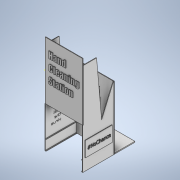
# Autodesk Inventor part: hand-cleaning-body
Saved by Autodesk Inventor 2020.2 (Build 242310000, 310)
## iProperties
Created: 2020-03-25
Part Number: hand-cleaning-body
Material: Generic
Document SubType Name: Modeling
Designer: iamin
Density: 1 g/cm^3
Appearance: Default
Author: iamin
Autodesk Inventor part; units mm, degrees
(part 1 of 2)
ref_plane "YZ Plane" through (0, 0, 0) normal (1, 0, 0) x (0, 1, 0)
ref_plane "XY Plane" through (0, 0, 0) normal (0, 0, 1) x (1, 0, 0)
sketch "Sketch1" plane through (0, 0, 0) normal (0, 0, 1) x (1, 0, 0)
  line L0 (-45.3, -70) -> (45.3, -70)
  line L1 (45.3, -70) -> (45.3, 70)
  line L2 (45.3, 70) -> (-45.3, 70)
  line L3 (-45.3, 70) -> (-45.3, -70)
  line L4 (-45.3, -70) -> (45.3, 70) construction
  line L5 (45.3, -70) -> (-45.3, 70) construction
  point P0 (0, 0)
  dimension "topsize" = 90.6
  dimension "d1" = 140
  constraints: 12 end point, 2 midpoint, 2 parallel, 1 horizontal, 1 perpendicular
  measures "topsize" distance of L2.end L1.end
  measures "d1" distance of L1.end L0.end
extrude "Extrusion1" add sketch "Sketch1" along normal mid plane 1.3
sketch "Sketch2" plane through (45.3, -70, 0.65) normal (1, 0, 0) x (0, 0, -1)
  line L0 (1.3, 125.1437) -> (33.3, 125.1437)
  line L1 (-0.1992, -99) -> (140.3032, -99)
  line L2 (1.3, 0) -> (0, 0) projected
  line L3 (75.8394, -99) -> (75.8394, 14.3341)
  line L4 (1.3, 140) -> (1.3, 0) projected
  line L5 (33.3, 125.1437) -> (45.5649, -11.2927)
  line L6 (74.2941, 54.8516) -> (45.5649, -11.2927)
  line L7 (75.8394, 14.3341) -> (75.8394, 54.8516)
  line L8 (75.8394, 54.8516) -> (74.2941, 54.8516)
  line L9 (-0.1992, 0) -> (-0.1992, -99)
  line L10 (0.65, 0) -> (-0.1992, 0)
  point P0 (0.65, 70)
  dimension "d4" = 99
  dimension "d5" = 74.5394
  dimension "d7" = 32
  constraints: 18 end point, 3 horizontal, 3 vertical, 2 point on line, 1 midpoint, 1 perpendicular
  measures "d4" distance between parallel lines of L1 L2
  measures "d5" distance from line of L3 L2.start
  measures "d7" distance of L0.start L0.end
extrude "Extrusion2" add sketch "Sketch2" along normal mid plane 1.3
mirror "Mirror1" about plane through (0, 0, 0) normal (1, 0, 0) of "Extrusion2"
sketch "Sketch3" plane through (-45.95, -169, -75.1894) normal (-1, 0, 0) x (0, 0, 1)
  point P0 (75.1894, 169)
sketch "Sketch4" plane through (45.95, -169, -75.1894) normal (0, 0, -1) x (-1, 0, 0)
  line L0 (-0.1836, 153.786) -> (91.9029, 153.786)
  line L1 (91.9029, 153.786) -> (91.9029, 0.1386)
  line L2 (91.9029, 0.1386) -> (-0.1836, 0.1386)
  line L3 (-0.1836, 0.1386) -> (-0.1836, 153.786)
  point P0 (45.95, 169)
  constraints: 8 end point, 2 parallel, 1 horizontal, 1 perpendicular
extrude "Extrusion3" add sketch "Sketch4" along normal mid plane 1.3
sketch "Sketch5" plane through (-45.95, -70, -0.65) normal (-1, 0, 0) x (0, 0, 1)
  line L0 (-75.2386, -98.82) -> (-124.9776, -98.82)
  line L1 (-75.2386, -96.5831) -> (-124.9776, -96.5831)
  line L2 (-124.9776, -96.5831) -> (-124.9776, -98.82)
  line L3 (-75.2386, -96.5831) -> (-75.2386, -98.82)
  point P0 (0.65, 70)
  constraints: 8 end point, 2 horizontal, 1 perpendicular, 1 vertical
extrude "Extrusion4" add sketch "Sketch5" against normal blind 91.9
sketch "Sketch6" plane through (-45.95, -70, -0.65) normal (-1, 0, 0) x (0, 0, 1)
  point P0 (0.65, 70)
sketch "Sketch7" plane through (-44.65, -169, 0.8492) normal (0, 0, 1) x (1, 0, 0)
  line L0 (0, 24.5) -> (1.5, 24.5)
  line L1 (1.5, 24.5) -> (1.5, 26)
  line L2 (1.5, 26) -> (0, 26)
  line L3 (0, 0) -> (1.5, 0)
  line L4 (1.5, 0) -> (1.5, 1.5)
  line L5 (1.5, 1.5) -> (0, 1.5)
  line L6 (0, 26) -> (0, 0)
  point P0 (44.65, 169)
  point P1 (0, 24.5)
  point P2 (0, 1.5)
  dimension "d15" = 1.5
  dimension "d16" = 1.5
  dimension "d17" = 1.5
  dimension "d18" = 1.5
  dimension "d19" = 26
  constraints: 14 end point, 4 perpendicular, 2 horizontal, 1 vertical
  measures "d15" distance of L0.start L0.end
  measures "d16" distance of L3.start L3.end
  measures "d17" distance of L3.end L4.end
  measures "d18" distance of L1.end L0.end
  measures "d19" distance of L1.end L3.end
extrude "Extrusion5" add sketch "Sketch7" against normal blind 74.5394
mirror "Mirror2" about plane through (0, 0, 0) normal (1, 0, 0) of "Extrusion5"
sketch "Sketch8" plane through (-44.65, -70, -0.65) normal (0, -1, 0) x (1, 0, 0)
  line L0 (0, 0) -> (44.65, 0)
  line L1 (44.65, -41.1247) -> (0, -41.1247)
  line L2 (0, -41.1247) -> (0, 0)
  line L3 (89.3, 0) -> (44.65, 0)
  line L4 (44.65, -41.1247) -> (89.3, -41.1247)
  line L5 (89.3, -41.1247) -> (89.3, 0)
  point P0 (44.65, 0.65)
  constraints: 12 end point, 1 horizontal, 1 parallel
extrude "Extrusion6" [suppressed]
sketch "Sketch10" plane through (-45.9529, -15.214, -75.8394) normal (0, 1, 0) x (1, 0, 0)
  line L0 (58.8396, -1.3) -> (58.8396, -5.46)
  line L1 (58.8396, -5.46) -> (55.5586, -5.46)
  line L2 (55.5586, -5.46) -> (55.5586, -4.16)
  line L3 (55.5586, -4.16) -> (57.5396, -4.16)
  line L4 (57.5396, -4.16) -> (57.5396, -1.3)
  line L5 (90.6029, -1.3) -> (1.3029, -1.3) projected
  line L6 (45.9529, 0.1482) -> (45.9529, -6.4647)
  line L7 (58.8396, -1.3) -> (57.5396, -1.3)
  line L8 (33.0662, -1.3) -> (33.0662, -5.46)
  line L9 (33.0662, -5.46) -> (36.3472, -5.46)
  line L10 (36.3472, -5.46) -> (36.3472, -4.16)
  line L11 (36.3472, -4.16) -> (34.3662, -4.16)
  line L12 (34.3662, -4.16) -> (34.3662, -1.3)
  line L13 (1.3029, -1.3) -> (90.6029, -1.3)
  line L14 (33.0662, -1.3) -> (34.3662, -1.3)
  point P0 (45.9529, -75.8394)
  dimension "d25" = 1.3
  dimension "d26" = 1.3
  dimension "d27" = 2.86
  constraints: 28 end point, 8 symmetric about line, 3 perpendicular, 2 horizontal, 2 vertical, 1 point on line
  measures "d25" distance between parallel lines of L0 L4
  measures "d26" distance between parallel lines of L1 L3
  measures "d27" distance between parallel lines of L5 L3
extrude "Extrusion7" [suppressed]
sketch "Sketch11" plane through (0, 0, 0.65) normal (0, 0, 1) x (1, 0, 0)
  line L0 (-36.7165, 46.3764) -> (38.2753, 46.3764) construction
  line L1 (38.2753, 46.3764) -> (38.2753, 2.6535) construction
  line L2 (38.2753, 2.6535) -> (-36.7165, 2.6535) construction
  line L3 (-36.7165, 2.6535) -> (-36.7165, 46.3764) construction
  line L4 (-26.2582, 46.3764) -> (-26.2582, 30.2764)
  line L5 (-26.2582, 30.2764) -> (-30.444, 30.2764)
  line L6 (-30.444, 30.2764) -> (-30.444, 37.0343)
  line L7 (-30.444, 37.0343) -> (-31.6936, 37.0343)
  line L8 (-31.6936, 37.0343) -> (-31.6936, 30.2764)
  line L9 (-31.6936, 30.2764) -> (-35.8794, 30.2764)
  line L10 (-35.8794, 30.2764) -> (-35.8794, 46.3764)
  line L11 (-35.8794, 46.3764) -> (-31.6936, 46.3764)
  line L12 (-31.6936, 46.3764) -> (-31.6936, 40.6134)
  line L13 (-31.6936, 40.6134) -> (-30.444, 40.6134)
  line L14 (-30.444, 40.6134) -> (-30.444, 46.3764)
  line L15 (-30.444, 46.3764) -> (-26.2582, 46.3764)
  line L16 (-21.1018, 38.3689) -> (-24.8751, 38.3689)
  line L17 (-24.8751, 38.3689) -> (-24.8751, 39.2546)
  spline S0 degree 2 poles (-24.8751, 39.2546) (-24.8751, 40.7833) (-24.1714, 42.4455) (-22.036, 43.7194) (-20.3375, 43.7194) knots 0 0 0 1 2 3 3 3
  spline S1 degree 2 poles (-20.3375, 43.7194) (-18.2992, 43.7194) (-16.2245, 42.2756) (-15.812, 40.1767) (-15.812, 36.9009) knots 0 0 0 1 2 3 3 3
  line L18 (-15.812, 36.9009) -> (-15.812, 30.2764)
  line L19 (-15.812, 30.2764) -> (-19.7187, 30.2764)
  line L20 (-19.7187, 30.2764) -> (-19.7187, 31.4533)
  spline S2 degree 2 poles (-19.7187, 31.4533) (-20.0827, 30.7496) (-21.2474, 30.0338) (-22.0603, 30.0338) knots 0 0 0 1 2 2 2
  spline S3 degree 2 poles (-22.0603, 30.0338) (-23.1158, 30.0338) (-24.8751, 31.2228) (-24.8751, 33.2247) knots 0 0 0 1 2 2 2
  line L21 (-24.8751, 33.2247) -> (-24.8751, 34.3045)
  spline S4 degree 2 poles (-24.8751, 34.3045) (-24.8751, 35.7847) (-23.9409, 36.8645) (-22.0846, 37.5803) knots 0 0 0 1 2 2 2
  spline S5 degree 2 poles (-22.0846, 37.5803) (-20.107, 38.3568) (-19.8279, 38.8906) (-19.8279, 39.7156) knots 0 0 0 1 2 2 2
  spline S6 degree 2 poles (-19.8279, 39.7156) (-19.8279, 40.7469) (-20.1312, 41.3778) (-20.4952, 41.3778) knots 0 0 0 1 2 2 2
  spline S7 degree 2 poles (-20.4952, 41.3778) (-20.9077, 41.3778) (-21.1018, 40.8561) (-21.1018, 39.752) knots 0 0 0 1 2 2 2
  line L22 (-21.1018, 39.752) -> (-21.1018, 38.3689)
  spline S8 degree 2 poles (-19.8279, 36.5612) (-20.7985, 35.8575) (-21.1018, 34.899) (-21.1018, 34.0012) knots 0 0 0 1 2 2 2
  spline S9 degree 2 poles (-21.1018, 34.0012) (-21.1018, 32.9699) (-20.8349, 32.3754) (-20.4345, 32.3754) knots 0 0 0 1 2 2 2
  spline S10 degree 2 poles (-20.4345, 32.3754) (-20.0584, 32.3754) (-19.8279, 32.8486) (-19.8279, 33.8434) knots 0 0 0 1 2 2 2
  line L23 (-19.8279, 33.8434) -> (-19.8279, 36.5612)
  line L24 (-10.3402, 43.4767) -> (-10.413, 42.2635)
  spline S11 degree 2 poles (-10.413, 42.2635) (-9.9762, 42.9914) (-8.7144, 43.7194) (-7.8894, 43.7194) knots 0 0 0 1 2 2 2
  spline S12 degree 2 poles (-7.8894, 43.7194) (-6.846, 43.7194) (-5.5357, 42.7488) (-5.1596, 41.2565) (-5.1596, 39.5336) knots 0 0 0 1 2 3 3 3
  line L25 (-5.1596, 39.5336) -> (-5.1596, 30.2764)
  line L26 (-5.1596, 30.2764) -> (-9.1755, 30.2764)
  line L27 (-9.1755, 30.2764) -> (-9.1755, 39.4123)
  spline S13 degree 2 poles (-9.1755, 39.4123) (-9.1755, 40.7833) (-9.3574, 41.3778) (-9.77, 41.3778) knots 0 0 0 1 2 2 2
  spline S14 degree 2 poles (-9.77, 41.3778) (-10.1946, 41.3778) (-10.413, 40.6862) (-10.413, 39.1939) knots 0 0 0 1 2 2 2
  line L28 (-10.413, 39.1939) -> (-10.413, 30.2764)
  line L29 (-10.413, 30.2764) -> (-14.4289, 30.2764)
  line L30 (-14.4289, 30.2764) -> (-14.4289, 43.4767)
  line L31 (-14.4289, 43.4767) -> (-10.3402, 43.4767)
  line L32 (5.3594, 46.3764) -> (5.3594, 30.2764)
  line L33 (5.3594, 30.2764) -> (1.3435, 30.2764)
  line L34 (1.3435, 30.2764) -> (1.3435, 31.2349)
  spline S15 degree 2 poles (1.3435, 31.2349) (0.7612, 30.6283) (-0.5006, 30.0338) (-1.2043, 30.0338) knots 0 0 0 1 2 2 2
  spline S16 degree 2 poles (-1.2043, 30.0338) (-2.1385, 30.0338) (-3.5095, 31.0165) (-3.8978, 32.3147) (-3.8978, 33.7706) knots 0 0 0 1 2 3 3 3
  line L35 (-3.8978, 33.7706) -> (-3.8978, 39.9583)
  spline S17 degree 2 poles (-3.8978, 39.9583) (-3.8978, 41.4749) (-3.5095, 42.7488) (-2.1143, 43.7194) (-1.1558, 43.7194) knots 0 0 0 1 2 3 3 3
  spline S18 degree 2 poles (-1.1558, 43.7194) (-0.4036, 43.7194) (0.834, 43.1856) (1.3435, 42.6396) knots 0 0 0 1 2 2 2
  line L36 (1.3435, 42.6396) -> (1.3435, 46.3764)
  line L37 (1.3435, 46.3764) -> (5.3594, 46.3764)
  spline S19 degree 2 poles (1.3435, 40.1524) (1.3435, 40.8804) (1.0888, 41.3778) (0.7248, 41.3778) knots 0 0 0 1 2 2 2
  spline S20 degree 2 poles (0.7248, 41.3778) (0.3729, 41.3778) (0.1181, 40.9289) (0.1181, 40.1524) knots 0 0 0 1 2 2 2
  line L38 (0.1181, 40.1524) -> (0.1181, 33.6857)
  spline S21 degree 2 poles (0.1181, 33.6857) (0.1181, 32.885) (0.3608, 32.3754) (0.7005, 32.3754) knots 0 0 0 1 2 2 2
  spline S22 degree 2 poles (0.7005, 32.3754) (1.0888, 32.3754) (1.3435, 32.9456) (1.3435, 34.0497) knots 0 0 0 1 2 2 2
  line L39 (1.3435, 34.0497) -> (1.3435, 40.1524)
  line L40 (-26.1005, 12.4203) -> (-30.2862, 12.4203)
  line L41 (-30.2862, 12.4203) -> (-30.2862, 15.2229)
  spline S23 degree 2 poles (-30.2862, 15.2229) (-30.2862, 16.4362) (-30.5531, 17.0428) (-31.0142, 17.0428) knots 0 0 0 1 2 2 2
  spline S24 degree 2 poles (-31.0142, 17.0428) (-31.5359, 17.0428) (-31.8149, 16.3027) (-31.8149, 15.0895) knots 0 0 0 1 2 2 2
  line L42 (-31.8149, 15.0895) -> (-31.8149, 7.6158)
  spline S25 degree 2 poles (-31.8149, 7.6158) (-31.8149, 6.4389) (-31.5359, 5.7231) (-31.0506, 5.7231) knots 0 0 0 1 2 2 2
  spline S26 degree 2 poles (-31.0506, 5.7231) (-30.5774, 5.7231) (-30.2862, 6.4389) (-30.2862, 7.7614) knots 0 0 0 1 2 2 2
  line L43 (-30.2862, 7.7614) -> (-30.2862, 9.7875)
  line L44 (-30.2862, 9.7875) -> (-26.1005, 9.7875)
  line L45 (-26.1005, 9.7875) -> (-26.1005, 9.1566)
  spline S27 degree 2 poles (-26.1005, 9.1566) (-26.1005, 6.6573) (-26.8042, 4.5705) (-29.2307, 2.9932) (-30.9899, 2.9932) knots 0 0 0 1 2 3 3 3
  spline S28 degree 2 poles (-30.9899, 2.9932) (-32.8341, 2.9932) (-35.2242, 4.3278) (-36.0007, 6.6816) (-36.0007, 9.0474) knots 0 0 0 1 2 3 3 3
  line L46 (-36.0007, 9.0474) -> (-36.0007, 13.7549)
  spline S29 degree 2 poles (-36.0007, 13.7549) (-36.0007, 15.4898) (-35.758, 17.2369) (-34.5812, 18.8506) (-32.4822, 19.7727) (-31.1112, 19.7727) knots 0 0 0 1 2 3 4 4 4
  spline S30 degree 2 poles (-31.1112, 19.7727) (-29.2671, 19.7727) (-26.8527, 18.341) (-26.1005, 16.2057) (-26.1005, 13.949) knots 0 0 0 1 2 3 3 3
  line L47 (-26.1005, 13.949) -> (-26.1005, 12.4203)
  line L48 (-20.5801, 19.4329) -> (-20.5801, 3.3329)
  line L49 (-20.5801, 3.3329) -> (-24.7174, 3.3329)
  line L50 (-24.7174, 3.3329) -> (-24.7174, 19.4329)
  line L51 (-24.7174, 19.4329) -> (-20.5801, 19.4329)
  line L52 (-10.0369, 9.7026) -> (-15.2418, 9.7026)
  line L53 (-15.2418, 9.7026) -> (-15.2418, 6.8514)
  spline S31 degree 2 poles (-15.2418, 6.8514) (-15.2418, 5.9536) (-14.987, 5.4319) (-14.6109, 5.4319) knots 0 0 0 1 2 2 2
  spline S32 degree 2 poles (-14.6109, 5.4319) (-14.1498, 5.4319) (-13.8465, 6.1235) (-13.8465, 7.1062) knots 0 0 0 1 2 2 2
  line L54 (-13.8465, 7.1062) -> (-13.8465, 8.8412)
  line L55 (-13.8465, 8.8412) -> (-10.0369, 8.8412)
  line L56 (-10.0369, 8.8412) -> (-10.0369, 7.8705)
  spline S33 degree 2 poles (-10.0369, 7.8705) (-10.0369, 6.6452) (-10.3402, 5.3348) (-11.4807, 3.8425) (-13.2156, 3.0903) (-14.5381, 3.0903) knots 0 0 0 1 2 3 4 4 4
  spline S34 degree 2 poles (-14.5381, 3.0903) (-15.812, 3.0903) (-17.7532, 3.8304) (-18.8452, 5.1164) (-19.2577, 6.6573) (-19.2577, 8.1253) knots 0 0 0 1 2 3 4 4 4
  line L57 (-19.2577, 8.1253) -> (-19.2577, 11.9835)
  spline S35 degree 2 poles (-19.2577, 11.9835) (-19.2577, 13.7063) (-18.3235, 15.7082) (-16.1881, 16.7759) (-14.8171, 16.7759) knots 0 0 0 1 2 3 3 3
  spline S36 degree 2 poles (-14.8171, 16.7759) (-13.1186, 16.7759) (-10.9226, 15.4898) (-10.0369, 13.3788) (-10.0369, 11.4497) knots 0 0 0 1 2 3 3 3
  line L58 (-10.0369, 11.4497) -> (-10.0369, 9.7026)
  line L59 (-14.0649, 11.8501) -> (-14.0649, 12.8085)
  spline S37 degree 2 poles (-14.0649, 12.8085) (-14.0649, 13.8398) (-14.2833, 14.4343) (-14.623, 14.4343) knots 0 0 0 1 2 2 2
  spline S38 degree 2 poles (-14.623, 14.4343) (-15.0476, 14.4343) (-15.2418, 13.9247) (-15.2418, 12.8085) knots 0 0 0 1 2 2 2
  line L60 (-15.2418, 12.8085) -> (-15.2418, 11.8501)
  line L61 (-15.2418, 11.8501) -> (-14.0649, 11.8501)
  line L62 (-5.1353, 11.4254) -> (-8.9085, 11.4254)
  line L63 (-8.9085, 11.4254) -> (-8.9085, 12.3111)
  spline S39 degree 2 poles (-8.9085, 12.3111) (-8.9085, 13.8398) (-8.2048, 15.502) (-6.0695, 16.7759) (-4.3709, 16.7759) knots 0 0 0 1 2 3 3 3
  spline S40 degree 2 poles (-4.3709, 16.7759) (-2.3327, 16.7759) (-0.258, 15.3321) (0.1545, 13.2332) (0.1545, 9.9574) knots 0 0 0 1 2 3 3 3
  line L64 (0.1545, 9.9574) -> (0.1545, 3.3329)
  line L65 (0.1545, 3.3329) -> (-3.7522, 3.3329)
  line L66 (-3.7522, 3.3329) -> (-3.7522, 4.5098)
  spline S41 degree 2 poles (-3.7522, 4.5098) (-4.1161, 3.8061) (-5.2809, 3.0903) (-6.0938, 3.0903) knots 0 0 0 1 2 2 2
  spline S42 degree 2 poles (-6.0938, 3.0903) (-7.1493, 3.0903) (-8.9085, 4.2793) (-8.9085, 6.2812) knots 0 0 0 1 2 2 2
  line L67 (-8.9085, 6.2812) -> (-8.9085, 7.361)
  spline S43 degree 2 poles (-8.9085, 7.361) (-8.9085, 8.8412) (-7.9743, 9.921) (-6.118, 10.6368) knots 0 0 0 1 2 2 2
  spline S44 degree 2 poles (-6.118, 10.6368) (-4.1404, 11.4133) (-3.8614, 11.9471) (-3.8614, 12.7721) knots 0 0 0 1 2 2 2
  spline S45 degree 2 poles (-3.8614, 12.7721) (-3.8614, 13.8034) (-4.1647, 14.4343) (-4.5287, 14.4343) knots 0 0 0 1 2 2 2
  spline S46 degree 2 poles (-4.5287, 14.4343) (-4.9412, 14.4343) (-5.1353, 13.9126) (-5.1353, 12.8085) knots 0 0 0 1 2 2 2
  line L68 (-5.1353, 12.8085) -> (-5.1353, 11.4254)
  spline S47 degree 2 poles (-3.8614, 9.6176) (-4.832, 8.914) (-5.1353, 7.9555) (-5.1353, 7.0577) knots 0 0 0 1 2 2 2
  spline S48 degree 2 poles (-5.1353, 7.0577) (-5.1353, 6.0264) (-4.8684, 5.4319) (-4.468, 5.4319) knots 0 0 0 1 2 2 2
  spline S49 degree 2 poles (-4.468, 5.4319) (-4.0919, 5.4319) (-3.8614, 5.9051) (-3.8614, 6.8999) knots 0 0 0 1 2 2 2
  line L69 (-3.8614, 6.8999) -> (-3.8614, 9.6176)
  line L70 (5.6264, 16.5332) -> (5.5536, 15.32)
  spline S50 degree 2 poles (5.5536, 15.32) (5.9903, 16.0479) (7.2521, 16.7759) (8.0771, 16.7759) knots 0 0 0 1 2 2 2
  spline S51 degree 2 poles (8.0771, 16.7759) (9.1206, 16.7759) (10.4309, 15.8053) (10.807, 14.313) (10.807, 12.5901) knots 0 0 0 1 2 3 3 3
  line L71 (10.807, 12.5901) -> (10.807, 3.3329)
  line L72 (10.807, 3.3329) -> (6.7911, 3.3329)
  line L73 (6.7911, 3.3329) -> (6.7911, 12.4688)
  spline S52 degree 2 poles (6.7911, 12.4688) (6.7911, 13.8398) (6.6091, 14.4343) (6.1966, 14.4343) knots 0 0 0 1 2 2 2
  spline S53 degree 2 poles (6.1966, 14.4343) (5.7719, 14.4343) (5.5536, 13.7427) (5.5536, 12.2504) knots 0 0 0 1 2 2 2
  line L74 (5.5536, 12.2504) -> (5.5536, 3.3329)
  line L75 (5.5536, 3.3329) -> (1.5377, 3.3329)
  line L76 (1.5377, 3.3329) -> (1.5377, 16.5332)
  line L77 (1.5377, 16.5332) -> (5.6264, 16.5332)
  line L78 (16.3273, 16.5332) -> (16.3273, 3.3329)
  line L79 (16.3273, 3.3329) -> (12.1901, 3.3329)
  line L80 (12.1901, 3.3329) -> (12.1901, 16.5332)
  line L81 (12.1901, 16.5332) -> (16.3273, 16.5332)
  line L82 (16.3273, 19.4329) -> (16.3273, 17.334)
  line L83 (16.3273, 17.334) -> (12.1901, 17.334)
  line L84 (12.1901, 17.334) -> (12.1901, 19.4329)
  line L85 (12.1901, 19.4329) -> (16.3273, 19.4329)
  line L86 (21.8598, 16.5332) -> (21.787, 15.32)
  spline S54 degree 2 poles (21.787, 15.32) (22.2238, 16.0479) (23.4856, 16.7759) (24.3106, 16.7759) knots 0 0 0 1 2 2 2
  spline S55 degree 2 poles (24.3106, 16.7759) (25.354, 16.7759) (26.6643, 15.8053) (27.0404, 14.313) (27.0404, 12.5901) knots 0 0 0 1 2 3 3 3
  line L87 (27.0404, 12.5901) -> (27.0404, 3.3329)
  line L88 (27.0404, 3.3329) -> (23.0245, 3.3329)
  line L89 (23.0245, 3.3329) -> (23.0245, 12.4688)
  spline S56 degree 2 poles (23.0245, 12.4688) (23.0245, 13.8398) (22.8426, 14.4343) (22.43, 14.4343) knots 0 0 0 1 2 2 2
  spline S57 degree 2 poles (22.43, 14.4343) (22.0054, 14.4343) (21.787, 13.7427) (21.787, 12.2504) knots 0 0 0 1 2 2 2
  line L90 (21.787, 12.2504) -> (21.787, 3.3329)
  line L91 (21.787, 3.3329) -> (17.7711, 3.3329)
  line L92 (17.7711, 3.3329) -> (17.7711, 16.5332)
  line L93 (17.7711, 16.5332) -> (21.8598, 16.5332)
  line L94 (37.5594, 16.5332) -> (37.5594, 6.3661)
  spline S58 degree 2 poles (37.5594, 6.3661) (37.5594, 4.3036) (37.3653, 3.1024) (36.2127, 1.7557) (34.1502, 1.052) (32.5972, 1.052) knots 0 0 0 1 2 3 4 4 4
  spline S59 degree 2 poles (32.5972, 1.052) (30.6681, 1.052) (28.3386, 2.3502) (28.3022, 4.2672) knots 0 0 0 1 2 2 2
  line L95 (28.3022, 4.2672) -> (32.1968, 4.2672)
  spline S60 degree 2 poles (32.1968, 4.2672) (32.1968, 3.3936) (32.8398, 3.3936) knots 0 0 0 1 1 1
  spline S61 degree 2 poles (32.8398, 3.3936) (33.3009, 3.3936) (33.6042, 3.9274) (33.6042, 4.7889) knots 0 0 0 1 2 2 2
  line L96 (33.6042, 4.7889) -> (33.6042, 5.7837)
  spline S62 degree 2 poles (33.6042, 5.7837) (33.0825, 5.3106) (31.942, 4.8374) (31.3111, 4.8374) knots 0 0 0 1 2 2 2
  spline S63 degree 2 poles (31.3111, 4.8374) (30.2313, 4.8374) (28.8239, 5.7109) (28.3022, 7.1305) (28.3022, 8.4529) knots 0 0 0 1 2 3 3 3
  line L97 (28.3022, 8.4529) -> (28.3022, 13.2453)
  spline S64 degree 2 poles (28.3022, 13.2453) (28.3022, 15.1259) (29.6611, 16.7759) (31.0442, 16.7759) knots 0 0 0 1 2 2 2
  spline S65 degree 2 poles (31.0442, 16.7759) (31.7964, 16.7759) (33.0461, 16.1571) (33.5314, 15.5384) knots 0 0 0 1 2 2 2
  line L98 (33.5314, 15.5384) -> (33.8226, 16.5332)
  line L99 (33.8226, 16.5332) -> (37.5594, 16.5332)
  spline S66 degree 2 poles (33.5314, 13.0269) (33.5314, 13.9369) (33.3251, 14.4343) (32.9612, 14.4343) knots 0 0 0 1 2 2 2
  spline S67 degree 2 poles (32.9612, 14.4343) (32.6093, 14.4343) (32.3181, 13.8641) (32.3181, 13.0269) knots 0 0 0 1 2 2 2
  line L100 (32.3181, 13.0269) -> (32.3181, 8.5864)
  spline S68 degree 2 poles (32.3181, 8.5864) (32.3181, 7.7007) (32.5365, 7.179) (32.8884, 7.179) knots 0 0 0 1 2 2 2
  spline S69 degree 2 poles (32.8884, 7.179) (33.2888, 7.179) (33.5314, 7.822) (33.5314, 8.9382) knots 0 0 0 1 2 2 2
  line L101 (33.5314, 8.9382) -> (33.5314, 13.0269)
  line L102 (-27.0104, -12.3757) -> (-30.905, -12.3757)
  line L103 (-30.905, -12.3757) -> (-30.905, -11.1867)
  spline S70 degree 2 poles (-30.905, -11.1867) (-30.905, -10.3617) (-31.1962, -9.9007) (-31.548, -9.9007) knots 0 0 0 1 2 2 2
  spline S71 degree 2 poles (-31.548, -9.9007) (-31.9241, -9.9007) (-32.3124, -10.5194) (-32.3124, -11.1382) knots 0 0 0 1 2 2 2
  spline S72 degree 2 poles (-32.3124, -11.1382) (-32.3124, -11.939) (-32.094, -12.3515) knots 0 0 0 1 1 1
  spline S73 degree 2 poles (-32.094, -12.3515) (-31.8756, -12.764) (-30.905, -13.3342) knots 0 0 0 1 1 1
  spline S74 degree 2 poles (-30.905, -13.3342) (-28.1145, -14.9964) (-27.3865, -16.0641) knots 0 0 0 1 1 1
  spline S75 degree 2 poles (-27.3865, -16.0641) (-26.6586, -17.1317) (-26.6586, -19.4976) knots 0 0 0 1 1 1
  spline S76 degree 2 poles (-26.6586, -19.4976) (-26.6586, -21.2204) (-27.4593, -22.8462) (-29.7767, -23.9503) (-31.3054, -23.9503) knots 0 0 0 1 2 3 3 3
  spline S77 degree 2 poles (-31.3054, -23.9503) (-32.9797, -23.9503) (-35.3577, -22.6763) (-36.0978, -20.7109) (-36.0978, -18.9031) knots 0 0 0 1 2 3 3 3
  line L104 (-36.0978, -18.9031) -> (-36.0978, -17.8476)
  line L105 (-36.0978, -17.8476) -> (-32.2032, -17.8476)
  line L106 (-32.2032, -17.8476) -> (-32.2032, -19.8009)
  spline S78 degree 2 poles (-32.2032, -19.8009) (-32.2032, -20.6987) (-31.8756, -21.2204) (-31.4631, -21.2204) knots 0 0 0 1 2 2 2
  spline S79 degree 2 poles (-31.4631, -21.2204) (-31.0385, -21.2204) (-30.6381, -20.5653) (-30.6381, -19.9222) knots 0 0 0 1 2 2 2
  spline S80 degree 2 poles (-30.6381, -19.9222) (-30.6381, -18.5027) (-31.0263, -18.0659) knots 0 0 0 1 1 1
  spline S81 degree 2 poles (-31.0263, -18.0659) (-31.4267, -17.6292) (-32.9918, -16.5979) knots 0 0 0 1 1 1
  spline S82 degree 2 poles (-32.9918, -16.5979) (-34.5448, -15.5666) (-35.5639, -14.6324) (-36.2312, -12.9824) (-36.2312, -11.6963) knots 0 0 0 1 2 3 3 3
  spline S83 degree 2 poles (-36.2312, -11.6963) (-36.2312, -9.84) (-35.2849, -8.1293) (-33.1738, -7.1708) (-31.6815, -7.1708) knots 0 0 0 1 2 3 3 3
  spline S84 degree 2 poles (-31.6815, -7.1708) (-30.0557, -7.1708) (-27.7505, -8.2264) (-27.0104, -9.8279) (-27.0104, -11.7448) knots 0 0 0 1 2 3 3 3
  line L107 (-27.0104, -11.7448) -> (-27.0104, -12.3757)
  line L108 (-21.2353, -8.651) -> (-21.2353, -10.7257)
  line L109 (-21.2353, -10.7257) -> (-20.1434, -10.7257)
  line L110 (-20.1434, -10.7257) -> (-20.1434, -12.8125)
  line L111 (-20.1434, -12.8125) -> (-21.2353, -12.8125)
  line L112 (-21.2353, -12.8125) -> (-21.2353, -19.8858)
  spline S85 degree 2 poles (-21.2353, -19.8858) (-21.2353, -21.184) (-20.9684, -21.4873) (-19.9735, -21.4873) knots 0 0 0 1 2 2 2
  line L113 (-19.9735, -21.4873) -> (-19.9735, -23.6106)
  line L114 (-19.9735, -23.6106) -> (-21.5993, -23.6106)
  spline S86 degree 2 poles (-21.5993, -23.6106) (-22.9703, -23.6106) (-24.1471, -23.38) (-25.0449, -22.555) (-25.2633, -21.4873) (-25.2633, -19.5219) knots 0 0 0 1 2 3 4 4 4
  line L115 (-25.2633, -19.5219) -> (-25.2633, -12.8125)
  line L116 (-25.2633, -12.8125) -> (-26.1247, -12.8125)
  line L117 (-26.1247, -12.8125) -> (-26.1247, -10.7257)
  line L118 (-26.1247, -10.7257) -> (-25.2633, -10.7257)
  line L119 (-25.2633, -10.7257) -> (-25.2633, -8.651)
  line L120 (-25.2633, -8.651) -> (-21.2353, -8.651)
  line L121 (-15.6664, -15.5181) -> (-19.4397, -15.5181)
  line L122 (-19.4397, -15.5181) -> (-19.4397, -14.6324)
  spline S87 degree 2 poles (-19.4397, -14.6324) (-19.4397, -13.1037) (-18.736, -11.4415) (-16.6006, -10.1676) (-14.9021, -10.1676) knots 0 0 0 1 2 3 3 3
  spline S88 degree 2 poles (-14.9021, -10.1676) (-12.8638, -10.1676) (-10.7891, -11.6114) (-10.3766, -13.7103) (-10.3766, -16.9861) knots 0 0 0 1 2 3 3 3
  line L123 (-10.3766, -16.9861) -> (-10.3766, -23.6106)
  line L124 (-10.3766, -23.6106) -> (-14.2833, -23.6106)
  line L125 (-14.2833, -23.6106) -> (-14.2833, -22.4337)
  spline S89 degree 2 poles (-14.2833, -22.4337) (-14.6473, -23.1374) (-15.812, -23.8532) (-16.6249, -23.8532) knots 0 0 0 1 2 2 2
  spline S90 degree 2 poles (-16.6249, -23.8532) (-17.6804, -23.8532) (-19.4397, -22.6642) (-19.4397, -20.6623) knots 0 0 0 1 2 2 2
  line L126 (-19.4397, -20.6623) -> (-19.4397, -19.5825)
  spline S91 degree 2 poles (-19.4397, -19.5825) (-19.4397, -18.1023) (-18.5054, -17.0225) (-16.6492, -16.3067) knots 0 0 0 1 2 2 2
  spline S92 degree 2 poles (-16.6492, -16.3067) (-14.6715, -15.5302) (-14.3925, -14.9964) (-14.3925, -14.1714) knots 0 0 0 1 2 2 2
  spline S93 degree 2 poles (-14.3925, -14.1714) (-14.3925, -13.1401) (-14.6958, -12.5092) (-15.0598, -12.5092) knots 0 0 0 1 2 2 2
  spline S94 degree 2 poles (-15.0598, -12.5092) (-15.4723, -12.5092) (-15.6664, -13.0309) (-15.6664, -14.135) knots 0 0 0 1 2 2 2
  line L127 (-15.6664, -14.135) -> (-15.6664, -15.5181)
  spline S95 degree 2 poles (-14.3925, -17.3259) (-15.3631, -18.0295) (-15.6664, -18.988) (-15.6664, -19.8858) knots 0 0 0 1 2 2 2
  spline S96 degree 2 poles (-15.6664, -19.8858) (-15.6664, -20.9171) (-15.3995, -21.5116) (-14.9991, -21.5116) knots 0 0 0 1 2 2 2
  spline S97 degree 2 poles (-14.9991, -21.5116) (-14.623, -21.5116) (-14.3925, -21.0384) (-14.3925, -20.0436) knots 0 0 0 1 2 2 2
  line L128 (-14.3925, -20.0436) -> (-14.3925, -17.3259)
  line L129 (-4.7592, -8.651) -> (-4.7592, -10.7257)
  line L130 (-4.7592, -10.7257) -> (-3.6672, -10.7257)
  line L131 (-3.6672, -10.7257) -> (-3.6672, -12.8125)
  line L132 (-3.6672, -12.8125) -> (-4.7592, -12.8125)
  line L133 (-4.7592, -12.8125) -> (-4.7592, -19.8858)
  spline S98 degree 2 poles (-4.7592, -19.8858) (-4.7592, -21.184) (-4.4923, -21.4873) (-3.4974, -21.4873) knots 0 0 0 1 2 2 2
  line L134 (-3.4974, -21.4873) -> (-3.4974, -23.6106)
  line L135 (-3.4974, -23.6106) -> (-5.1232, -23.6106)
  spline S99 degree 2 poles (-5.1232, -23.6106) (-6.4941, -23.6106) (-7.671, -23.38) (-8.5688, -22.555) (-8.7872, -21.4873) (-8.7872, -19.5219) knots 0 0 0 1 2 3 4 4 4
  line L136 (-8.7872, -19.5219) -> (-8.7872, -12.8125)
  line L137 (-8.7872, -12.8125) -> (-9.6486, -12.8125)
  line L138 (-9.6486, -12.8125) -> (-9.6486, -10.7257)
  line L139 (-9.6486, -10.7257) -> (-8.7872, -10.7257)
  line L140 (-8.7872, -10.7257) -> (-8.7872, -8.651)
  line L141 (-8.7872, -8.651) -> (-4.7592, -8.651)
  line L142 (1.3557, -10.4103) -> (1.3557, -23.6106)
  line L143 (1.3557, -23.6106) -> (-2.7816, -23.6106)
  line L144 (-2.7816, -23.6106) -> (-2.7816, -10.4103)
  line L145 (-2.7816, -10.4103) -> (1.3557, -10.4103)
  line L146 (1.3557, -7.5106) -> (1.3557, -9.6095)
  line L147 (1.3557, -9.6095) -> (-2.7816, -9.6095)
  line L148 (-2.7816, -9.6095) -> (-2.7816, -7.5106)
  line L149 (-2.7816, -7.5106) -> (1.3557, -7.5106)
  line L150 (11.8868, -15.0449) -> (11.8868, -18.2843)
  spline S100 degree 2 poles (11.8868, -18.2843) (11.8868, -20.0557) (11.5349, -21.7179) (10.3581, -23.1616) (8.5139, -23.8532) (7.3249, -23.8532) knots 0 0 0 1 2 3 4 4 4
  spline S101 degree 2 poles (7.3249, -23.8532) (5.9903, -23.8532) (4.134, -23.2708) (3.1149, -22.0818) (2.6781, -20.3954) (2.6781, -18.7211) knots 0 0 0 1 2 3 4 4 4
  line L151 (2.6781, -18.7211) -> (2.6781, -15.3361)
  spline S102 degree 2 poles (2.6781, -15.3361) (2.6781, -13.4919) (3.4789, -11.4173) (5.5414, -10.1676) (7.1551, -10.1676) knots 0 0 0 1 2 3 3 3
  spline S103 degree 2 poles (7.1551, -10.1676) (8.5018, -10.1676) (10.443, -10.9684) (11.4985, -12.2665) (11.8868, -13.6375) (11.8868, -15.0449) knots 0 0 0 1 2 3 4 4 4
  spline S104 degree 2 poles (7.8709, -14.05) (7.8709, -13.0309) (7.6525, -12.5092) (7.2885, -12.5092) knots 0 0 0 1 2 2 2
  spline S105 degree 2 poles (7.2885, -12.5092) (6.9367, -12.5092) (6.694, -13.0309) (6.694, -14.05) knots 0 0 0 1 2 2 2
  line L152 (6.694, -14.05) -> (6.694, -20.0072)
  spline S106 degree 2 poles (6.694, -20.0072) (6.694, -20.9414) (6.9367, -21.5116) (7.2885, -21.5116) knots 0 0 0 1 2 2 2
  spline S107 degree 2 poles (7.2885, -21.5116) (7.6404, -21.5116) (7.8709, -20.9899) (7.8709, -20.1406) knots 0 0 0 1 2 2 2
  line L153 (7.8709, -20.1406) -> (7.8709, -14.05)
  line L154 (17.2979, -10.4103) -> (17.2251, -11.6235)
  spline S108 degree 2 poles (17.2251, -11.6235) (17.6619, -10.8956) (18.9237, -10.1676) (19.7487, -10.1676) knots 0 0 0 1 2 2 2
  spline S109 degree 2 poles (19.7487, -10.1676) (20.7921, -10.1676) (22.1025, -11.1382) (22.4786, -12.6305) (22.4786, -14.3534) knots 0 0 0 1 2 3 3 3
  line L155 (22.4786, -14.3534) -> (22.4786, -23.6106)
  line L156 (22.4786, -23.6106) -> (18.4627, -23.6106)
  line L157 (18.4627, -23.6106) -> (18.4627, -14.4747)
  spline S110 degree 2 poles (18.4627, -14.4747) (18.4627, -13.1037) (18.2807, -12.5092) (17.8682, -12.5092) knots 0 0 0 1 2 2 2
  spline S111 degree 2 poles (17.8682, -12.5092) (17.4435, -12.5092) (17.2251, -13.2008) (17.2251, -14.6931) knots 0 0 0 1 2 2 2
  line L158 (17.2251, -14.6931) -> (17.2251, -23.6106)
  line L159 (17.2251, -23.6106) -> (13.2092, -23.6106)
  line L160 (13.2092, -23.6106) -> (13.2092, -10.4103)
  line L161 (13.2092, -10.4103) -> (17.2979, -10.4103)
  point P0 (0, 0)
  constraints: 2 other
extrude "Extrusion8" add sketch "Sketch11" against normal mid plane 2.6
sketch "Sketch12" plane through (-45.95, -70, -0.65) normal (-1, 0, 0) x (0, 0, 1)
  line L0 (-37.1355, -25.1951) -> (-11.1638, -25.1951) construction
  line L1 (-11.1638, -25.1951) -> (-11.1638, -28.7149) construction
  line L2 (-11.1638, -28.7149) -> (-37.1355, -28.7149) construction
  line L3 (-37.1355, -28.7149) -> (-37.1355, -25.1951) construction
  line L4 (-36.1668, -29.0652) -> (-35.2604, -29.0652)
  line L5 (-35.2604, -29.0652) -> (-35.2604, -27.2524)
  line L6 (-35.2604, -27.2524) -> (-36.1668, -27.2524)
  line L7 (-36.1668, -27.2524) -> (-36.1668, -27.123)
  line L8 (-36.1668, -27.123) -> (-35.2604, -27.123)
  line L9 (-35.2604, -27.123) -> (-35.2604, -25.2431)
  line L10 (-35.2604, -25.2431) -> (-35.1309, -25.2431)
  line L11 (-35.1309, -25.2431) -> (-35.1309, -27.123)
  line L12 (-35.1309, -27.123) -> (-33.3182, -27.123)
  line L13 (-33.3182, -27.123) -> (-33.3182, -25.2431)
  line L14 (-33.3182, -25.2431) -> (-33.1887, -25.2431)
  line L15 (-33.1887, -25.2431) -> (-33.1887, -27.123)
  line L16 (-33.1887, -27.123) -> (-32.2823, -27.123)
  line L17 (-32.2823, -27.123) -> (-32.2823, -27.2524)
  line L18 (-32.2823, -27.2524) -> (-33.1887, -27.2524)
  line L19 (-33.1887, -27.2524) -> (-33.1887, -29.0652)
  line L20 (-33.1887, -29.0652) -> (-32.2823, -29.0652)
  line L21 (-32.2823, -29.0652) -> (-32.2823, -29.1947)
  line L22 (-32.2823, -29.1947) -> (-33.1887, -29.1947)
  line L23 (-33.1887, -29.1947) -> (-33.1887, -31.0697)
  line L24 (-33.1887, -31.0697) -> (-33.3182, -31.0697)
  line L25 (-33.3182, -31.0697) -> (-33.3182, -29.1947)
  line L26 (-33.3182, -29.1947) -> (-35.1309, -29.1947)
  line L27 (-35.1309, -29.1947) -> (-35.1309, -31.0697)
  line L28 (-35.1309, -31.0697) -> (-35.2604, -31.0697)
  line L29 (-35.2604, -31.0697) -> (-35.2604, -29.1947)
  line L30 (-35.2604, -29.1947) -> (-36.1668, -29.1947)
  line L31 (-36.1668, -29.1947) -> (-36.1668, -29.0652)
  line L32 (-35.1309, -29.0652) -> (-33.3182, -29.0652)
  line L33 (-33.3182, -29.0652) -> (-33.3182, -27.2524)
  line L34 (-33.3182, -27.2524) -> (-35.1309, -27.2524)
  line L35 (-35.1309, -27.2524) -> (-35.1309, -29.0652)
  line L36 (-30.3977, -31.0697) -> (-30.3977, -25.2431)
  line L37 (-30.3977, -25.2431) -> (-30.2682, -25.2431)
  line L38 (-30.2682, -25.2431) -> (-30.2682, -28.0917)
  line L39 (-30.2682, -28.0917) -> (-29.3858, -28.0917)
  line L40 (-29.3858, -28.0917) -> (-26.4988, -25.1951)
  line L41 (-26.4988, -25.1951) -> (-26.4029, -25.291)
  line L42 (-26.4029, -25.291) -> (-29.2707, -28.154)
  line L43 (-29.2707, -28.154) -> (-26.4029, -31.0218)
  line L44 (-26.4029, -31.0218) -> (-26.4988, -31.1177)
  line L45 (-26.4988, -31.1177) -> (-29.3858, -28.2211)
  line L46 (-29.3858, -28.2211) -> (-30.2682, -28.2211)
  line L47 (-30.2682, -28.2211) -> (-30.2682, -31.0697)
  line L48 (-30.2682, -31.0697) -> (-30.3977, -31.0697)
  line L49 (-24.5758, -31.0697) -> (-24.5758, -27.1853)
  line L50 (-24.5758, -27.1853) -> (-24.4463, -27.1853)
  line L51 (-24.4463, -27.1853) -> (-24.4463, -31.0697)
  line L52 (-24.4463, -31.0697) -> (-24.5758, -31.0697)
  line L53 (-24.5758, -26.2118) -> (-24.5758, -25.2431)
  line L54 (-24.5758, -25.2431) -> (-24.4463, -25.2431)
  line L55 (-24.4463, -25.2431) -> (-24.4463, -26.2118)
  line L56 (-24.4463, -26.2118) -> (-24.5758, -26.2118)
  line L57 (-21.6409, -31.1177) -> (-22.6288, -30.1202)
  line L58 (-22.6288, -30.1202) -> (-22.6288, -25.2431)
  line L59 (-22.6288, -25.2431) -> (-22.4993, -25.2431)
  line L60 (-22.4993, -25.2431) -> (-22.4993, -30.0722)
  line L61 (-22.4993, -30.0722) -> (-21.545, -31.0218)
  line L62 (-21.545, -31.0218) -> (-21.6409, -31.1177)
  line L63 (-18.73, -31.1177) -> (-19.7179, -30.1202)
  line L64 (-19.7179, -30.1202) -> (-19.7179, -25.2431)
  line L65 (-19.7179, -25.2431) -> (-19.5884, -25.2431)
  line L66 (-19.5884, -25.2431) -> (-19.5884, -30.0722)
  line L67 (-19.5884, -30.0722) -> (-18.6341, -31.0218)
  line L68 (-18.6341, -31.0218) -> (-18.73, -31.1177)
  line L69 (-32.2344, -40.7771) -> (-33.2558, -41.789)
  line L70 (-33.2558, -41.789) -> (-34.2917, -40.7531)
  line L71 (-34.2917, -40.7531) -> (-34.2917, -37.8806)
  line L72 (-34.2917, -37.8806) -> (-36.1668, -37.8806)
  line L73 (-36.1668, -37.8806) -> (-36.1668, -37.7511)
  line L74 (-36.1668, -37.7511) -> (-34.2917, -37.7511)
  line L75 (-34.2917, -37.7511) -> (-34.2917, -35.8712)
  line L76 (-34.2917, -35.8712) -> (-34.1622, -35.8712)
  line L77 (-34.1622, -35.8712) -> (-34.1622, -37.7511)
  line L78 (-34.1622, -37.7511) -> (-32.2871, -37.7511)
  line L79 (-32.2871, -37.7511) -> (-32.2871, -37.8806)
  line L80 (-32.2871, -37.8806) -> (-34.1622, -37.8806)
  line L81 (-34.1622, -37.8806) -> (-34.1622, -40.7052)
  line L82 (-34.1622, -40.7052) -> (-33.2558, -41.6067)
  line L83 (-33.2558, -41.6067) -> (-32.3303, -40.6764)
  line L84 (-32.3303, -40.6764) -> (-32.2344, -40.7771)
  line L85 (-30.4024, -41.6979) -> (-30.4024, -35.8712)
  line L86 (-30.4024, -35.8712) -> (-30.273, -35.8712)
  line L87 (-30.273, -35.8712) -> (-30.273, -39.6022)
  line L88 (-30.273, -39.6022) -> (-28.4219, -37.7511)
  line L89 (-28.4219, -37.7511) -> (-27.4004, -37.7511)
  line L90 (-27.4004, -37.7511) -> (-26.3885, -38.763)
  line L91 (-26.3885, -38.763) -> (-26.3885, -41.6979)
  line L92 (-26.3885, -41.6979) -> (-26.518, -41.6979)
  line L93 (-26.518, -41.6979) -> (-26.518, -38.8109)
  line L94 (-26.518, -38.8109) -> (-27.4484, -37.8806)
  line L95 (-27.4484, -37.8806) -> (-28.3691, -37.8806)
  line L96 (-28.3691, -37.8806) -> (-30.273, -39.7796)
  line L97 (-30.273, -39.7796) -> (-30.273, -41.6979)
  line L98 (-30.273, -41.6979) -> (-30.4024, -41.6979)
  line L99 (-21.5977, -41.765) -> (-23.5639, -41.765)
  line L100 (-23.5639, -41.765) -> (-24.5758, -40.7531)
  line L101 (-24.5758, -40.7531) -> (-24.5758, -38.763)
  line L102 (-24.5758, -38.763) -> (-23.5639, -37.7511)
  line L103 (-23.5639, -37.7511) -> (-21.5738, -37.7511)
  line L104 (-21.5738, -37.7511) -> (-20.5379, -38.7869)
  line L105 (-20.5379, -38.7869) -> (-21.5738, -39.8228)
  line L106 (-21.5738, -39.8228) -> (-24.4463, -39.8228)
  line L107 (-24.4463, -39.8228) -> (-24.4463, -40.7052)
  line L108 (-24.4463, -40.7052) -> (-23.516, -41.6355)
  line L109 (-23.516, -41.6355) -> (-21.5977, -41.6355)
  line L110 (-21.5977, -41.6355) -> (-21.5977, -41.765)
  line L111 (-24.4463, -39.6933) -> (-21.6217, -39.6933)
  line L112 (-21.6217, -39.6933) -> (-20.7153, -38.7869)
  line L113 (-20.7153, -38.7869) -> (-21.6217, -37.8806)
  line L114 (-21.6217, -37.8806) -> (-23.516, -37.8806)
  line L115 (-23.516, -37.8806) -> (-24.4463, -38.8109)
  line L116 (-24.4463, -38.8109) -> (-24.4463, -39.6933)
  line L117 (-32.2248, -48.4703) -> (-34.2197, -52.4699)
  line L118 (-34.2197, -52.4699) -> (-36.2195, -48.4703)
  line L119 (-36.2195, -48.4703) -> (-36.1044, -48.408)
  line L120 (-36.1044, -48.408) -> (-34.2197, -52.1821)
  line L121 (-34.2197, -52.1821) -> (-32.3351, -48.408)
  line L122 (-32.3351, -48.408) -> (-32.2248, -48.4703)
  line L123 (-30.4024, -52.326) -> (-30.4024, -48.4416)
  line L124 (-30.4024, -48.4416) -> (-30.273, -48.4416)
  line L125 (-30.273, -48.4416) -> (-30.273, -52.326)
  line L126 (-30.273, -52.326) -> (-30.4024, -52.326)
  line L127 (-30.4024, -47.4681) -> (-30.4024, -46.4993)
  line L128 (-30.4024, -46.4993) -> (-30.273, -46.4993)
  line L129 (-30.273, -46.4993) -> (-30.273, -47.4681)
  line L130 (-30.273, -47.4681) -> (-30.4024, -47.4681)
  line L131 (-28.4554, -52.326) -> (-28.4554, -48.4416)
  line L132 (-28.4554, -48.4416) -> (-28.326, -48.4416)
  line L133 (-28.326, -48.4416) -> (-28.326, -50.2303)
  line L134 (-28.326, -50.2303) -> (-26.4749, -48.3792)
  line L135 (-26.4749, -48.3792) -> (-25.4534, -48.3792)
  line L136 (-25.4534, -48.3792) -> (-24.4607, -49.3671)
  line L137 (-24.4607, -49.3671) -> (-24.5566, -49.463)
  line L138 (-24.5566, -49.463) -> (-25.5013, -48.5087)
  line L139 (-25.5013, -48.5087) -> (-26.4269, -48.5087)
  line L140 (-26.4269, -48.5087) -> (-28.326, -50.4078)
  line L141 (-28.326, -50.4078) -> (-28.326, -52.326)
  line L142 (-28.326, -52.326) -> (-28.4554, -52.326)
  line L143 (-18.7491, -50.5372) -> (-20.6002, -52.3931)
  line L144 (-20.6002, -52.3931) -> (-21.6217, -52.3931)
  line L145 (-21.6217, -52.3931) -> (-22.6336, -51.3813)
  line L146 (-22.6336, -51.3813) -> (-22.6336, -48.4416)
  line L147 (-22.6336, -48.4416) -> (-22.5041, -48.4416)
  line L148 (-22.5041, -48.4416) -> (-22.5041, -51.3333)
  line L149 (-22.5041, -51.3333) -> (-21.5738, -52.2637)
  line L150 (-21.5738, -52.2637) -> (-20.653, -52.2637)
  line L151 (-20.653, -52.2637) -> (-18.7491, -50.3598)
  line L152 (-18.7491, -50.3598) -> (-18.7491, -48.4416)
  line L153 (-18.7491, -48.4416) -> (-18.6197, -48.4416)
  line L154 (-18.6197, -48.4416) -> (-18.6197, -52.326)
  line L155 (-18.6197, -52.326) -> (-18.7491, -52.326)
  line L156 (-18.7491, -52.326) -> (-18.7491, -50.5372)
  line L157 (-16.7398, -52.2637) -> (-13.8528, -52.2637)
  line L158 (-13.8528, -52.2637) -> (-12.9465, -51.3573)
  line L159 (-12.9465, -51.3573) -> (-13.8528, -50.4509)
  line L160 (-13.8528, -50.4509) -> (-15.7951, -50.4509)
  line L161 (-15.7951, -50.4509) -> (-16.8309, -49.4151)
  line L162 (-16.8309, -49.4151) -> (-15.7951, -48.3792)
  line L163 (-15.7951, -48.3792) -> (-12.8602, -48.3792)
  line L164 (-12.8602, -48.3792) -> (-12.8602, -48.5087)
  line L165 (-12.8602, -48.5087) -> (-15.7471, -48.5087)
  line L166 (-15.7471, -48.5087) -> (-16.6535, -49.4151)
  line L167 (-16.6535, -49.4151) -> (-15.7471, -50.3214)
  line L168 (-15.7471, -50.3214) -> (-13.8049, -50.3214)
  line L169 (-13.8049, -50.3214) -> (-12.769, -51.3573)
  line L170 (-12.769, -51.3573) -> (-13.8049, -52.3931)
  line L171 (-13.8049, -52.3931) -> (-16.7398, -52.3931)
  line L172 (-16.7398, -52.3931) -> (-16.7398, -52.2637)
  point P0 (0.65, 70)
  constraints: 2 other
extrude "Extrusion9" cut sketch "Sketch12" against normal blind 10